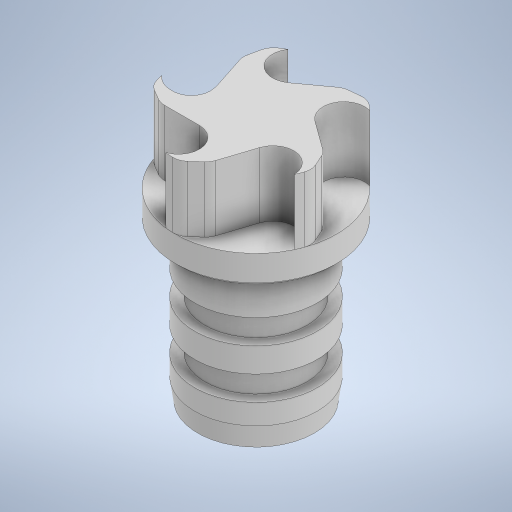
# Autodesk Inventor part: 4mm_uncorrected
Saved by Autodesk Inventor 2023.1 (Build 271208000, 208)
## iProperties
Created: 2021-06-23
Part Number: 4mm_uncorrected
Material: Generic
Document SubType Name: Modeling
Designer: student
Density: 1 g/cm^3
Appearance: Default
Author: student
Autodesk Inventor part; units mm, degrees
ref_plane "YZ Plane" through (0, 0, 0) normal (1, 0, 0) x (0, 1, 0)
sketch "Sketch1" plane through (0, 0, 0) normal (0, 1, 0) x (-1, 0, 0)
  line L0 (-0.649, -1.6053) -> (-0.9398, -1.6357)
  line L1 (-0.419, 1.6799) -> (-0.2016, 1.8756)
  line L2 (-0.419, 1.6799) -> (-0.2016, 1.8756)
  arc A0 (0.9477, -1.7326) -> (0.2288, -1.0309) centre (0.5282, -1.4432) ccw
  line L3 (-0.4651, -1.5348) -> (0.2288, -1.0309)
  arc A1 (-1.355, -1.4369) -> (-1.2156, -1.5566) centre (-0.0001, 0.0001) ccw
  line L4 (-0.4651, -1.5348) -> (0.2288, -1.0309)
  arc A2 (-0.649, -1.6053) -> (-0.4651, -1.5348) centre (-0.6886, -1.227) ccw
  arc A3 (0.2515, 1.959) -> (0.4208, 0.9687) centre (0.4209, 1.4783) ccw
  line L5 (1.2782, 0.9685) -> (0.4208, 0.9687)
  arc A4 (1.4685, 0.9175) -> (1.2782, 0.9685) centre (1.2781, 0.5882) ccw
  line L6 (1.4685, 0.9175) -> (1.7216, 0.7711)
  arc A5 (1.9407, 0.3661) -> (1.0503, -0.0998) centre (1.535, 0.0576) ccw
  line L7 (1.3158, -0.9173) -> (1.0503, -0.0998)
  arc A6 (1.326, -1.1141) -> (1.3158, -0.9173) centre (0.954, -1.0348) ccw
  line L8 (1.326, -1.1141) -> (1.2652, -1.3991)
  arc A7 (-1.7854, 0.8447) -> (-0.7912, 0.6997) centre (-1.2759, 0.8573) ccw
  line L9 (-0.5262, 1.5149) -> (-0.7912, 0.6997)
  arc A8 (-0.419, 1.6799) -> (-0.5262, 1.5149) centre (-0.1645, 1.3973) ccw
  line L10 (-1.7275, 0.1211) -> (-1.8462, 0.3883)
  arc A9 (-1.7275, 0.1211) -> (-1.6035, -0.0321) centre (-1.3799, 0.2756) ccw
  line L11 (-1.6035, -0.0321) -> (-0.9099, -0.5362)
  arc A10 (-1.355, -1.4369) -> (-0.9099, -0.5362) centre (-1.2095, -0.9485) ccw
  arc A11 (1.9407, 0.366) -> (1.8983, 0.5449) centre (-0.0001, 0.0001) ccw
  arc A12 (-1.7854, 0.8447) -> (-1.8562, 0.675) centre (-0.0001, 0.0001) ccw
  arc A13 (0.9477, -1.7326) -> (1.1047, -1.637) centre (-0.0001, 0.0001) ccw
  arc A14 (0.2515, 1.959) -> (0.0682, 1.9739) centre (-0.0001, 0.0001) ccw
  arc A15 (0.0682, 1.9739) -> (-0.2016, 1.8756) centre (0.0549, 1.5907) ccw
  arc A16 (-1.8562, 0.675) -> (-1.8462, 0.3883) centre (-1.4958, 0.544) ccw
  arc A17 (1.8983, 0.5449) -> (1.7216, 0.7711) centre (1.5297, 0.4392) ccw
  arc A18 (-1.2156, -1.5566) -> (-0.9398, -1.6357) centre (-0.9797, -1.2544) ccw
  arc A19 (1.1047, -1.637) -> (1.2652, -1.3991) centre (0.8902, -1.3192) ccw
  circle A20 centre (-0.0001, 0.0001) radius 1.975
  arc A21 (1.5271, 0.5672) -> (1.0286, 0.0001) centre (1.4772, 0.1085) ccw
  line L12 (1.7216, 0.7711) -> (1.4685, 0.9175)
  line L13 (1.0286, 0.9686) -> (0.615, 0.9686)
  arc A22 (-1.5257, 0.4131) -> (-0.7912, 0.6997) centre (-1.2759, 0.8573) ccw
  arc A23 (-0.0001, 1.1912) -> (0.4206, 0.9684) centre (0.3627, 1.3676) ccw
  line L14 (-0.419, 1.6799) -> (-0.2016, 1.8756)
  arc A24 (-0.7912, 0.6997) -> (-0.7912, 0.6997) centre (-1.0986, 0.7997) ccw
  line L15 (1.326, -1.1141) -> (1.2652, -1.3991)
  arc A25 (0.7729, -0.9962) -> (0.2288, -1.0309) centre (0.5282, -1.4432) ccw
  arc A26 (-0.9715, -1.3991) -> (-0.9099, -0.5362) centre (-1.2095, -0.9485) ccw
  line L16 (-1.0986, -0.3991) -> (-1.4958, -0.1103)
  line L17 (-0.649, -1.6053) -> (-0.9099, -1.6326)
  arc A27 (-1.7278, 0.1218) -> (-1.8462, 0.3883) centre (-12657.1556, -5624.5961) ccw
  arc A28 (1.9228, 0.3883) -> (1.5271, 0.5672) centre (1.535, 0.0576) ccw
  arc A29 (0.9477, -1.7326) -> (0.7509, -0.9848) centre (0.5282, -1.4432) ccw
  arc A30 (-1.3317, -1.4432) -> (-0.9715, -1.3991) centre (-1.2095, -0.9485) ccw
  arc A31 (0.2515, 1.959) -> (-0.0001, 1.1912) centre (0.603, 1.4187) ccw
  arc A32 (-1.7854, 0.8447) -> (-1.5257, 0.4131) centre (-1.2759, 0.8573) ccw
  point P0 (0, 0)
  point P1 (1.2784, 0.9684)
  point P2 (1.1047, -1.637)
  point P3 (1.9407, 0.3661)
  point P4 (1.8983, 0.5449)
  point P5 (0.0682, 1.9739)
  point P6 (-1.7854, 0.8447)
  point P7 (-1.8562, 0.675)
  point P8 (-1.355, -1.4369)
  point P9 (-1.2156, -1.5566)
  dimension "d0" = 3.95
  constraints: 89 point on circle, 36 end point, 33 centre point, 32 tangent, 17 equal radius, 5 collinear, 5 point on line, 3 concentric, 2 coincident
  measures "d0" diameter of A20
extrude "Extrusion1" add sketch "Sketch1" along normal blind 1.6 contours L0 A18 A1 A10 L11 A9 L10 A16 A12 A7 L9 A8 L1 A15 A14 A3 A23 L5 A4 L6 A17 A11 A5 A21 L7 A6 L8 A19 A13 A0 L3 A2 | A3 A23
sketch "Sketch2" plane through (0, 0, 0) normal (0, -1, 0) x (1, 0, 0)
  circle A0 centre (0, 0) radius 1.975
  dimension "d3" = 3.95
  constraints: 1 centre point, 1 coincident
  measures "d3" diameter of A0
extrude "Extrusion2" add sketch "Sketch2" along normal blind 0.7
sketch "Sketch3" plane through (0, -0.7, 0) normal (0, -1, 0) x (1, 0, 0)
  circle A0 centre (0, 0) radius 1.5
  circle A1 centre (0, 0) radius 0.85
  dimension "d6" = 3
  dimension "d7" = 1.7
  constraints: 2 centre point, 2 coincident
  measures "d6" diameter of A0
  measures "d7" diameter of A1
extrude "Extrusion3" add sketch "Sketch3" along normal blind 3.8
chamfer "Chamfer1" distance 0.5 angle 8 1 edges at (-1.5, -4.5, 0) measured on face at (1.4951, -3.2333, -0.1207)
ref_plane "Work Plane1" through (0, -3.5, 0) normal (0, -1, 0) x (1, 0, 0)
sketch "Sketch6" plane through (0, -3.5, 0) normal (0, -1, 0) x (1, 0, 0)
  circle A0 centre (0, 0) radius 1.25
  circle A1 centre (0, 0) radius 1.8158
  circle A2 centre (0, 0) radius 1.5 projected
  dimension "d22" = 0.25
  constraints: 2 centre point, 2 coincident
  measures "d22" radial gap between concentric circles of A2 A0
extrude "Extrusion5" cut sketch "Sketch6" against normal blind 0.6 contours A1 | A2
ref_plane "Work Plane2" through (0, -2, 0) normal (0, -1, 0) x (1, 0, 0)
sketch "Sketch12" plane through (0, -2, 0) normal (0, -1, 0) x (1, 0, 0)
  circle A0 centre (0, 0) radius 1.25
  circle A1 centre (0, 0) radius 1.5 projected
  circle A2 centre (0, 0) radius 1.6718
  dimension "d32" = 0.25
  constraints: 2 centre point, 2 coincident
  measures "d32" radial gap between concentric circles of A1 A0
extrude "Extrusion8" cut sketch "Sketch12" against normal mid plane 0.6 contours A1 | A2
chamfer "Chanfrein3" distance 0.075 angle 45 1 edges at (-1.975, -0.7, 0)
body "Solid1"
